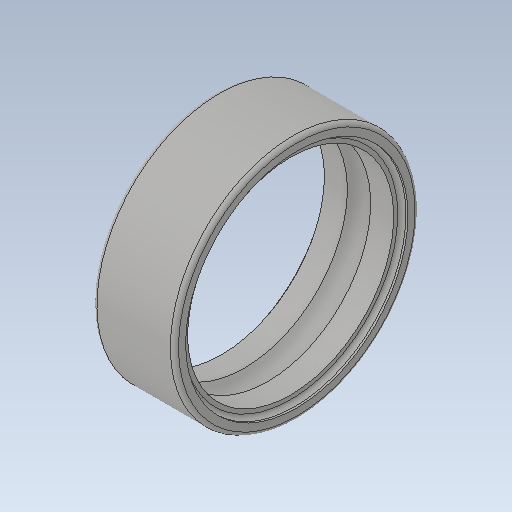
# Autodesk Inventor part: SKF_WBB1-8706-2RS1_PART2
Saved by Autodesk Inventor 2022 (Build 260153000, 153)
## iProperties
Created: 2022-10-07
Part Number: SKF_WBB1-8706-2RS1_PART2
Material: Generic
Catalog Web Link: www.cadenas.de
Description: -Deep groove ball bearings
Vendor: SKF
Document SubType Name: Modeling
Designer: psAdmin
Manufacturer: SKF
Mass: 2 g
Surface Area: 3.38303 cm^2
Volume: 0.117698 cm^3
Density: 1 g/cm^3
Appearance: PSOLRGB-175-175-175
Category: PARTsolutions
Company: SKF
PSOL_IDENT_0: {$CADENAS_DATA/23d-libs/skf/bearings_units_and_housings/ball_bearings/deep_groove_ball_bearings/bb1_
PSOL_IDENT_1: 001_101.prj},215 {VTYP=3D},{NB=SKF_WBB1-8706-2RS1_PART2},{LINA=SKF_WBB1-8706-2RS1_PART2},{NN=BB1_001
PSOL_IDENT_2: _101_PART2},{NOPRJ=TRUE},{DATE=09.09.2022 10:31:03},{GEOMDATE=07.09.2022 12:28:28},{VERSION=},{LINEI
PSOL_IDENT_3: D=21220},{WBVAR=},{WBNUMERIC=}  {NB=SKF_WBB1-8706-2RS1_PART2},{LINA=SKF_WBB1-8706-2RS1_PART2},{KT=DU
PSOL_IDENT_4: MMY},{DESIGNATION=WBB1-8706-2RS1},{R12=0.20},{DD=6.000},{D=12.000},{B=4.000},{C=},{CX=},{CXX=},{CA=0
PSOL_IDENT_5: .000},{XXVARIANT=},{XXDESIGN=Single row stainless steel},{XXSEALING=Contact seal on both sides},{DES
PSOL_IDENT_6: IGN=dgbb2rs},{DESIGNIR=dgbb2rs},{VARIANT=},{DD1=7.73},{DD2=7.2},{DD2X=},{DD2A=7.20},{D1=10.19},{D1X=
PSOL_IDENT_7: 0.00},{D2=10.9},{D2A=10.90},{D3=},{D3X=},{D3A=0.000},{D4=},{HH=0.000},{BB=0.000},{BBX=},{BBA=0.000},
PSOL_IDENT_8: {FF=},{R0MAX=0.000},{R0=0.000},{PITCH=9.00},{DW=1.588},{DDAMIN=7.100},{DDAMAX=7.100},{DDBMIN=0.000},
PSOL_IDENT_9: {DDBMAX=0.000},{DBMIN=0.000},{DAMAX=10.900},{BBAMIN=0.000},{CAMAX=0.000},{RAMAX=0.200},{LOAD1=0.403}
PSOL_IDENT_10: ,{LOAD2=0.146},{LOAD3=0.006},{SPEED1=0},{SPEED2=32000},{KR=0.015},{F0=7.400},{Z=8},{II=1},{MASS=0.00
PSOL_IDENT_11: 2},{BEARING=WBB1-8706-2RS1},{RING=},{HELP=0.905},{HELP2=0.550},{DD1ALG=3.865},{YALG=3.865},{PITCH1=9
PSOL_IDENT_12: .000},{DW1=1.588},{YALG1=5.095},{HALG1=0.905},{SH=3.600},{CU=0.482},{HALG=0.865},{B1=0},{SHIELDHELP=
PSOL_IDENT_13: 2},{D4A=0.000},{FFA=0.000},{RS1=},{HELP3=0},{SUPPRESS=0}
NB: SKF_WBB1-8706-2RS1_PART2
NT: Deep groove ball bearings
NBSYN: SKF_$DESIGNATION._PART2
LINA: SKF_WBB1-8706-2RS1_PART2
CATALOG: SKF
DESIGNATION: WBB1-8706-2RS1
R12: 0.2
DD: 6
D: 12
B: 4
XXDESIGN: Single row stainless steel
XXSEALING: Contact seal on both sides
DD2: 7.2
D2: 10.9
LOAD1: 0.403
LOAD2: 0.146
LOAD3: 0.006
SPEED1: 0
SPEED2: 32000
BEARING: WBB1-8706-2RS1
SUPPLIER: SKF
ARTICLENO: SKF_WBB1-8706-2RS1_PART2
BOMINFO: SKF_WBB1-8706-2RS1_PART2
CREATOR: CADENAS GmbH
Title: SKF_WBB1-8706-2RS1_PART2
Author: Cadenas PARTsolutions
Comments: Deep groove ball bearings
Autodesk Inventor part; units mm, degrees
ref_plane "YZ Plane" through (0, 0, 0) normal (1, 0, 0) x (0, 1, 0)
ref_plane "XZ Plane" through (0, 0, 0) normal (0, 1, 0) x (-1, 0, 0)
ref_plane "XY Plane" through (0, 0, 0) normal (0, 0, 1) x (1, 0, 0)
sketch "Sketch_9" plane through (0, 0, 0) normal (0, 0, 1) x (1, 0, 0)
  line L0 (50, 0) -> (-50, 0)
  line L1 (0, 5.8) -> (0, 5.45)
  line L2 (0, 5.45) -> (0.1, 5.45)
  arc A0 (0.3, 5.25) -> (0.1, 5.45) centre (0.1, 5.25) ccw
  line L3 (0.3, 5.25) -> (0.3, 5.05)
  line L4 (0.3, 5.05) -> (1.4273, 5.05)
  arc A1 (2.5727, 5.05) -> (1.4273, 5.05) centre (2, 4.5) ccw
  line L5 (2.5727, 5.05) -> (3.7, 5.05)
  line L6 (3.7, 5.05) -> (3.7, 5.25)
  arc A2 (3.9, 5.45) -> (3.7, 5.25) centre (3.9, 5.25) ccw
  line L7 (3.9, 5.45) -> (4, 5.45)
  line L8 (4, 5.45) -> (4, 5.8)
  arc A3 (4, 5.8) -> (3.8, 6) centre (3.8, 5.8) ccw
  line L9 (3.8, 6) -> (0.2, 6)
  arc A4 (0.2, 6) -> (0, 5.8) centre (0.2, 5.8) ccw
  constraints: 20 end point, 10 point on circle, 5 centre point
revolve "Revolution1" add sketch "Sketch_9" angle 360 about axis through (50, 0, 0) along (1, 0, 0)
body "Solid1"
